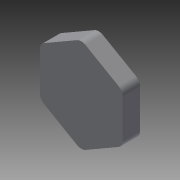
# Autodesk Inventor part: Nut
Saved by Autodesk Inventor 2014 SP1 (Build 180222100, 222)
## iProperties
Created: 2013-12-31
Part Number: Nut
Material: Generic
Document SubType Name: Modeling
Designer: tom
Density: 1 g/cm^3
Appearance: Default
Author: tom
Autodesk Inventor part; units mm, degrees
ref_plane "YZ Plane" through (0, 0, 0) normal (1, 0, 0) x (0, 1, 0)
ref_plane "XZ Plane" through (0, 0, 0) normal (0, 1, 0) x (-1, 0, 0)
ref_plane "XY Plane" through (0, 0, 0) normal (0, 0, 1) x (1, 0, 0)
sketch "Sketch1" plane through (0, 0, 0) normal (0, 0, 1) x (1, 0, 0)
  line L0 (0.5, 5.4848) -> (4.5, 3.1754)
  line L1 (5, 2.3094) -> (5, -2.3094)
  line L2 (4.5, -3.1754) -> (0.5, -5.4848)
  line L3 (-0.5, -5.4848) -> (-4.5, -3.1754)
  line L4 (-5, -2.3094) -> (-5, 2.3094)
  line L5 (-4.5, 3.1754) -> (-0.5, 5.4848)
  arc A0 (0.5, 5.4848) -> (-0.5, 5.4848) centre (0, 4.6188) ccw
  arc A1 (-4.5, 3.1754) -> (-5, 2.3094) centre (-4, 2.3094) ccw
  arc A2 (-5, -2.3094) -> (-4.5, -3.1754) centre (-4, -2.3094) ccw
  arc A3 (-0.5, -5.4848) -> (0.5, -5.4848) centre (0, -4.6188) ccw
  arc A4 (4.5, -3.1754) -> (5, -2.3094) centre (4, -2.3094) ccw
  arc A5 (5, 2.3094) -> (4.5, 3.1754) centre (4, 2.3094) ccw
  circle A6 centre (0, 0) radius 2.5
  point P0 (0, 5.7735)
  point P1 (5, 2.8868)
  point P2 (5, -2.8868)
  point P3 (0, -5.7735)
  point P4 (-5, -2.8868)
  point P5 (-5, 2.8868)
  dimension "d0" = 5
  dimension "d1" = 1
  dimension "d2" = 1
  dimension "d5" = 5
  constraints: 12 end point, 12 point on circle, 12 point on line, 12 tangent, 7 centre point, 4 equal radius, 2 coincident, 13 other
  measures "d0" distance from line of L0 point (0, 0)
  measures "d1" radius of A0
  measures "d2" radius of A1
  measures "d5" diameter of A6
extrude "Extrusion2" add sketch "Sketch1" along normal blind 2.1
body "Solid2"
